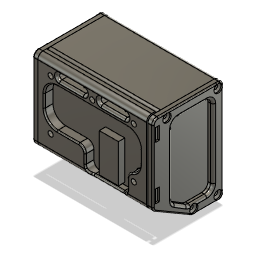
ToolheadExtensionsV2_Type_B v9 (Autodesk Fusion 360 design; units mm, degrees)
Autodesk Fusion 360 part; units mm, degrees
note: some values were not read from the file. Set by a fixed rule: which sketch regions a step uses.
sketch "Sketch1" plane through (0, 0, 0) normal (1, 0, 0) x (0, 0, -1) in component "Head"
  line L0 (0, 0) -> (0, 80)
  line L1 (0, 0) -> (-24, 0)
  line L2 (0, 80) -> (-48, 80)
  line L3 (-48, 80) -> (-48, 14)
  line L4 (-48, 14) -> (-24, 0)
  dimension "d1" = 80
  dimension "d2" = 24
  dimension "d3" = 48
  dimension "d4" = 66
  constraint coincident L0.start L1.start
  constraint vertical L0
  constraint perpendicular L0 L1
  constraint perpendicular L0 L2
  constraint perpendicular L2 L3
  measures "d1" distance of L0.start L0.end
  measures "d2" distance of L0.start L1.end
  measures "d3" distance of L0.end L2.end
  measures "d4" distance of L2.end L3.end
extrude "Extrude1" add sketch "Sketch1" along normal blind 86 makes body 1 in component "Head"
fillet "Fillet1" radius 3 5 edges at (43, 14, 48) (43, 0, 24) (43, 0, 0) (43, 80, 48) (43, 80, 0) on bodies 1 in component "Head"
sketch "Sketch2" plane through (0, 0, 0) normal (-1, 0, 0) x (0, 0, 1) in component "Head"
  arc A0 (3, 80) -> (0, 77) centre (3, 77) ccw
  line L0 (0, 77) -> (0, 3)
  arc A1 (0, 3) -> (3, 0) centre (3, 3) ccw
  line L1 (3, 0) -> (23.188953, 0)
  arc A2 (23.188953, 0) -> (24.700566, 0.408663) centre (23.188953, 3) ccw
  line L2 (24.700566, 0.408663) -> (46.511613, 13.131774)
  arc A3 (46.511613, 13.131774) -> (48, 15.723111) centre (45, 15.723111) ccw
  line L3 (48, 15.723111) -> (48, 77)
  arc A4 (48, 77) -> (45, 80) centre (45, 77) ccw
  line L4 (45, 80) -> (3, 80)
  line L5 (3, 77) -> (4, 77)
  line L6 (4, 77) -> (4, 76)
  line L7 (4, 76) -> (3, 76)
  line L8 (3, 76) -> (3, 77)
  line L9 (4, 76) -> (44, 76)
  line L10 (45, 77) -> (44, 77)
  line L11 (44, 77) -> (44, 76)
  line L12 (44, 76) -> (45, 76)
  line L13 (45, 76) -> (45, 77)
  line L14 (3, 3) -> (4, 3)
  line L15 (4, 3) -> (4, 4)
  line L16 (4, 4) -> (3, 4)
  line L17 (3, 4) -> (3, 3)
  line L18 (4, 4) -> (4, 76)
  line L19 (4, 4) -> (23, 4)
  line L20 (44, 76) -> (44, 16)
  circle A5 centre (4, 76) radius 1.5
  circle A6 centre (44, 76) radius 1.5
  circle A7 centre (23, 4) radius 1.5
  circle A8 centre (4, 4) radius 1.5
  dimension "d11" = 1
  dimension "d12" = 1
  dimension "d13" = 40
  dimension "d14" = 1
  dimension "d15" = 1
  dimension "d16" = 19
  dimension "d17" = 60
  dimension "d18" = 3
  dimension "d19" = 3
  dimension "d21" = 3
  dimension "d22" = 3
  constraint horizontal L5
  constraint vertical L6
  constraint horizontal L7
  constraint vertical L8
  constraint coincident A0.centre L5.start
  constraint perpendicular L6 L9
  constraint horizontal L10
  constraint vertical L11
  constraint horizontal L12
  constraint vertical L13
  constraint coincident A4.centre L10.start
  constraint horizontal L14
  constraint vertical L15
  constraint horizontal L16
  constraint vertical L17
  constraint coincident A1.centre L14.start
  constraint perpendicular L15 L19
  constraint perpendicular L9 L20
  constraint coincident L6.end L7.start
  constraint coincident L9.end L11.end
  constraint coincident L19.end A7.centre
  constraint coincident L15.end L16.start
  measures "d11" distance of A0.centre L5.end
  measures "d12" distance of A0.centre L7.end
  measures "d13" distance of L6.end L9.end
  measures "d14" distance of A1.centre L14.end
  measures "d15" distance of A1.centre L16.end
  measures "d16" distance of L15.end L19.end
  measures "d17" distance of L9.end L20.end
  measures "d18" diameter of A5
  measures "d19" diameter of A6
  measures "d21" diameter of A7
  measures "d22" diameter of A8
extrude "Extrude2" cut sketch "Sketch2" against normal blind 86 contours L9 L18 A5 | L9 L18 A5 | L5 L6 L7 L8 | L10 L11 L12 L13 | L9 L20 A6 | L9 L20 A6 | L14 L15 L16 L17 | L18 L19 A8 | L18 L19 A8 | A7 picked at (4.370476, 76.669113) picked at (4.875443, 75.521972) picked at (3.666667, 76.333333) picked at (44.333333, 76.333333) picked at (44.660764, 75.622125) picked at (43.065438, 75.651426) picked at (3.333333, 3.666667) picked at (4.370476, 3.330887) picked at (4.705305, 4.705305) picked at (22.804781, 5.044492) bodies 1 in component "Head"
sketch "Sketch1 (2)" plane through (0, 0, 0) normal (-1, 0, 0) x (0, 0, 1) in component "SideLeft"
  circle A0 centre (4, 4) radius 1.5
  circle A1 centre (44, 76) radius 1.5
  circle A2 centre (23, 4) radius 1.5
  circle A3 centre (4, 76) radius 1.5
  arc A4 (3, 80) -> (0, 77) centre (3, 77) ccw
  line L0 (0, 77) -> (0, 3)
  arc A5 (0, 3) -> (3, 0) centre (3, 3) ccw
  line L1 (3, 0) -> (23.188953, 0)
  arc A6 (23.188953, 0) -> (24.700566, 0.408663) centre (23.188953, 3) ccw
  line L2 (24.700566, 0.408663) -> (46.511613, 13.131774)
  arc A7 (46.511613, 13.131774) -> (48, 15.723111) centre (45, 15.723111) ccw
  line L3 (48, 15.723111) -> (48, 77)
  arc A8 (48, 77) -> (45, 80) centre (45, 77) ccw
  line L4 (45, 80) -> (3, 80)
  line L5 (4, 76) -> (8, 76)
  line L6 (8, 76) -> (8, 72)
  line L7 (8, 72) -> (4, 72)
  line L8 (4, 72) -> (4, 76)
  line L9 (44, 76) -> (40, 76)
  line L10 (40, 76) -> (40, 72)
  line L11 (40, 72) -> (44, 72)
  line L12 (44, 72) -> (44, 76)
  line L13 (4, 4) -> (8, 4)
  line L14 (8, 4) -> (8, 8)
  line L15 (8, 8) -> (4, 8)
  line L16 (4, 8) -> (4, 4)
  line L17 (23, 4) -> (23, 8)
  line L18 (44, 16) -> (40, 16)
  line L19 (29.797244, 3.381726) -> (27.10325, 8)
  line L20 (27.10325, 8) -> (40, 16)
  line L21 (40, 72) -> (40, 16)
  line L22 (27.10325, 8) -> (23, 8)
  line L23 (23, 8) -> (8, 8)
  line L24 (8, 72) -> (8, 8)
  line L25 (8, 72) -> (40, 72)
  dimension "d33" = 4
  dimension "d34" = 4
  dimension "d35" = 4
  dimension "d36" = 4
  dimension "d37" = 4
  dimension "d38" = 4
  dimension "d39" = 4
  dimension "d40" = 4
  constraint horizontal L5
  constraint vertical L6
  constraint horizontal L7
  constraint vertical L8
  constraint coincident A3.centre L5.start
  constraint horizontal L9
  constraint vertical L10
  constraint horizontal L11
  constraint vertical L12
  constraint coincident A1.centre L9.start
  constraint horizontal L13
  constraint vertical L14
  constraint horizontal L15
  constraint vertical L16
  constraint coincident A0.centre L13.start
  constraint coincident A2.centre L17.start
  constraint vertical L17
  constraint horizontal L18
  constraint perpendicular L2 L19
  constraint perpendicular L21 L22
  measures "d33" distance of A3.centre L5.end
  measures "d34" distance of A3.centre L7.end
  measures "d35" distance of A1.centre L9.end
  measures "d36" distance of A1.centre L11.end
  measures "d37" distance of A0.centre L13.end
  measures "d38" distance of A0.centre L15.end
  measures "d39" distance of A2.centre L17.end
  measures "d40" distance of L18.start L18.end
extrude "Extrude1'" add sketch "Sketch1 (2)" along normal blind 4 separate body contours A3 L5 L6 L7 L8 | A1 L9 L10 L11 L12 | A0 L13 L14 L15 L16 | A4 L0 A5 L1 A6 L2 A7 L3 A8 L4 picked at (7.087293, 74.396346) picked at (42.396346, 72.912707) picked at (7.087293, 5.603654) picked at (44, 34.57437) makes body 2 in component "SideLeft"
fillet "Fillet1'" radius 5 5 edges at (-2, 8, 8) (-2, 8, 27.10325) (-2, 16, 40) (-2, 72, 40) (-2, 72, 8) on bodies 2 in component "SideLeft"
hole "Hole1" at (-4, 76, 4) direction (1, 0, 0) diameter 6.5 depth 1 tip angle 118 bodies 2 in component "SideLeft"
hole "Hole2" at (-4, 76, 44) direction (1, 0, 0) diameter 6.5 depth 1 tip angle 118 bodies 2 in component "SideLeft"
hole "Hole4" at (-4, 4, 23) direction (1, 0, 0) diameter 6.5 depth 1 tip angle 118 bodies 2 in component "SideLeft"
hole "Hole5" at (-4, 4, 4) direction (1, 0, 0) diameter 6.5 depth 1 tip angle 118 bodies 2 in component "SideLeft"
sketch "Sketch2 (2)" plane through (-4, 0, 0) normal (-1, 0, 0) x (0, 0, 1) in component "SideLeft"
  circle A0 centre (4, 4) radius 3.25
  circle A1 centre (23, 4) radius 3.25
  circle A2 centre (44, 76) radius 3.25
  circle A3 centre (4, 76) radius 3.25
  line L0 (37.635654, 14.533369) -> (28.31406, 8.751079)
  arc A4 (25.678406, 8) -> (28.31406, 8.751079) centre (25.678406, 13) ccw
  line L1 (25.678406, 8) -> (13, 8)
  arc A5 (8, 13) -> (13, 8) centre (13, 13) ccw
  line L2 (8, 13) -> (8, 67)
  arc A6 (13, 72) -> (8, 67) centre (13, 67) ccw
  line L3 (13, 72) -> (35, 72)
  arc A7 (40, 67) -> (35, 72) centre (35, 67) ccw
  line L4 (40, 67) -> (40, 18.78229)
  arc A8 (37.635654, 14.533369) -> (40, 18.78229) centre (35, 18.78229) ccw
  line L5 (45, 80) -> (3, 80)
  arc A9 (3, 80) -> (0, 77) centre (3, 77) ccw
  line L6 (0, 77) -> (0, 3)
  arc A10 (0, 3) -> (3, 0) centre (3, 3) ccw
  line L7 (3, 0) -> (23.188953, 0)
  arc A11 (23.188953, 0) -> (24.700566, 0.408663) centre (23.188953, 3) ccw
  line L8 (24.700566, 0.408663) -> (46.511613, 13.131774)
  arc A12 (46.511613, 13.131774) -> (48, 15.723111) centre (45, 15.723111) ccw
  line L9 (48, 15.723111) -> (48, 77)
  arc A13 (48, 77) -> (45, 80) centre (45, 77) ccw
  line L10 (45, 80) -> (55, 80)
  line L11 (46.511613, 13.131774) -> (55, 18.083333)
  line L12 (55, 18.083333) -> (55, 80)
  dimension "d60" = 10
  constraint coincident L5.start A13.end
  constraint perpendicular L9 L10
  constraint tangent A12 L11
  constraint perpendicular L10 L12
  measures "d60" distance of L5.start L10.end
extrude "Extrude2'" add sketch "Sketch2 (2)" against normal blind 4 contours A12 L9 A13 L10 L11 L12 picked at (52.666667, 58.361111) bodies 2 in component "SideLeft"
fillet "Fillet2" radius 4 2 edges at (-2, 80, 55) (-2, 18.083333, 55) on bodies 2 in component "SideLeft"
sketch "Sketch3" plane through (-4, 0, 0) normal (-1, 0, 0) x (0, 0, 1) in component "SideLeft"
  circle A0 centre (4, 4) radius 3.25
  circle A1 centre (23, 4) radius 3.25
  circle A2 centre (44, 76) radius 3.25
  circle A3 centre (4, 76) radius 3.25
  line L0 (37.635654, 14.533369) -> (28.31406, 8.751079)
  arc A4 (25.678406, 8) -> (28.31406, 8.751079) centre (25.678406, 13) ccw
  line L1 (25.678406, 8) -> (13, 8)
  arc A5 (8, 13) -> (13, 8) centre (13, 13) ccw
  line L2 (8, 13) -> (8, 67)
  arc A6 (13, 72) -> (8, 67) centre (13, 67) ccw
  line L3 (13, 72) -> (35, 72)
  arc A7 (40, 67) -> (35, 72) centre (35, 67) ccw
  line L4 (40, 67) -> (40, 18.78229)
  arc A8 (37.635654, 14.533369) -> (40, 18.78229) centre (35, 18.78229) ccw
  arc A9 (53.015484, 16.925699) -> (55, 20.380815) centre (51, 20.380815) ccw
  line L5 (55, 20.380815) -> (55, 76)
  arc A10 (55, 76) -> (51, 80) centre (51, 76) ccw
  line L6 (51, 80) -> (3, 80)
  arc A11 (3, 80) -> (0, 77) centre (3, 77) ccw
  line L7 (0, 77) -> (0, 3)
  arc A12 (0, 3) -> (3, 0) centre (3, 3) ccw
  line L8 (3, 0) -> (23.188953, 0)
  arc A13 (23.188953, 0) -> (24.700566, 0.408663) centre (23.188953, 3) ccw
  line L9 (24.700566, 0.408663) -> (53.015484, 16.925699)
  line L10 (55, 76) -> (53, 76)
  line L11 (53, 76) -> (53, 74)
  line L12 (53, 74) -> (55, 74)
  line L13 (55, 74) -> (55, 76)
  line L14 (53, 74) -> (50, 74)
  line L15 (50, 74) -> (50, 64)
  line L16 (50, 64) -> (53, 64)
  line L17 (53, 64) -> (53, 74)
  line L18 (55, 20.380815) -> (53, 20.380815)
  line L19 (53, 20.380815) -> (53, 22.380815)
  line L20 (53, 22.380815) -> (55, 22.380815)
  line L21 (55, 22.380815) -> (55, 20.380815)
  line L22 (53, 22.380815) -> (50, 22.380815)
  line L23 (50, 22.380815) -> (50, 32.380815)
  line L24 (50, 32.380815) -> (53, 32.380815)
  line L25 (53, 32.380815) -> (53, 22.380815)
  dimension "d65" = 2
  dimension "d66" = 2
  dimension "d67" = 3
  dimension "d68" = 10
  dimension "d69" = 2
  dimension "d70" = 2
  dimension "d71" = 3
  dimension "d72" = 10
  constraint horizontal L10
  constraint vertical L11
  constraint horizontal L12
  constraint vertical L13
  constraint coincident L5.end A10.start
  constraint horizontal L14
  constraint vertical L15
  constraint horizontal L16
  constraint vertical L17
  constraint horizontal L18
  constraint vertical L19
  constraint horizontal L20
  constraint vertical L21
  constraint horizontal L22
  constraint vertical L23
  constraint horizontal L24
  constraint vertical L25
  measures "d65" distance of L5.end L10.end
  measures "d66" distance of L5.end L12.end
  measures "d67" distance of L11.end L14.end
  measures "d68" distance of L11.end L16.end
extrude "Extrude3" cut sketch "Sketch3" against normal blind 4 contours L22 L23 L24 L25 | L14 L15 L16 L17 picked at (51, 25.714148) picked at (51, 67.333333) bodies 2 in component "SideLeft"
fillet "Fillet4" radius 2 10 edges at (-4, 70.535534, 9.464466) (-4, 72, 24) (-4, 70.535534, 38.535534) (-4, 42.891145, 40) (-4, 16.351063, 39.369111) (-4, 11.642224, 32.974857) (-4, 8.191434, 27.048698) (-4, 8, 19.339203) (-4, 9.464466, 9.464466) (-4, 40, 8) on bodies 2 in component "SideLeft"
fillet "Fillet5" radius 1 10 edges at (-4, 78.828427, 53.828427) (-4, 80, 27) (-4, 79.12132, 0.87868) (-4, 40, 0) (-4, 0.87868, 0.87868) (-4, 0, 13.094476) (-4, 0.103967, 23.971893) (-4, 8.667181, 38.858025) (-4, 18.388572, 54.468569) (-4, 48.190407, 55) on bodies 2 in component "SideLeft"
ref_plane "WorkPlane1" through (43, 40, 24) normal (1, 0, 0) x (0, 0, -1)
mirror "MirrorComponent1" about plane through (0, 0, 0) normal (0, 0, 1) of bodies 2 makes body 3 in component "SideLeft(Mirror)"
sketch "Sketch1 (3)" plane through (0, 0, 0) normal (1, 0, 0) x (0, 0, -1) in component "Front_A"
  line L0 (-53, 74) -> (-50, 74)
  line L1 (-50, 74) -> (-50, 64)
  line L2 (-50, 64) -> (-53, 64)
  line L3 (-53, 64) -> (-53, 74)
  line L4 (-50, 32.380815) -> (-50, 22.380815)
  line L5 (-50, 22.380815) -> (-53, 22.380815)
  line L6 (-53, 22.380815) -> (-53, 32.380815)
  line L7 (-53, 32.380815) -> (-50, 32.380815)
  arc A0 (-55, 20.380815) -> (-53.015484, 16.925699) centre (-51, 20.380815) ccw
  line L8 (-53.015484, 16.925699) -> (-24.700566, 0.408663)
  arc A1 (-24.700566, 0.408663) -> (-23.188953, 0) centre (-23.188953, 3) ccw
  line L9 (-23.188953, 0) -> (-3, 0)
  arc A2 (-3, 0) -> (0, 3) centre (-3, 3) ccw
  line L10 (0, 3) -> (0, 77)
  arc A3 (0, 77) -> (-3, 80) centre (-3, 77) ccw
  line L11 (-3, 80) -> (-51, 80)
  arc A4 (-51, 80) -> (-55, 76) centre (-51, 76) ccw
  line L12 (-55, 76) -> (-55, 20.380815)
  circle A5 centre (-4, 76) radius 1.5
  arc A6 (-40, 18.78229) -> (-37.635654, 14.533369) centre (-35, 18.78229) ccw
  line L13 (-40, 18.78229) -> (-40, 67)
  arc A7 (-35, 72) -> (-40, 67) centre (-35, 67) ccw
  line L14 (-35, 72) -> (-13, 72)
  arc A8 (-8, 67) -> (-13, 72) centre (-13, 67) ccw
  line L15 (-8, 67) -> (-8, 13)
  arc A9 (-13, 8) -> (-8, 13) centre (-13, 13) ccw
  line L16 (-13, 8) -> (-25.678406, 8)
  arc A10 (-28.31406, 8.751079) -> (-25.678406, 8) centre (-25.678406, 13) ccw
  line L17 (-28.31406, 8.751079) -> (-37.635654, 14.533369)
  circle A11 centre (-44, 76) radius 1.5
  circle A12 centre (-23, 4) radius 1.5
  circle A13 centre (-4, 4) radius 1.5
  line L18 (-51, 80) -> (-48, 80)
  line L19 (-48, 80) -> (-48, 14)
  dimension "d75" = 3
  constraint coincident L11.end A4.start
  constraint parallel L11 L18
  constraint coincident L8 L19.end
  constraint perpendicular L18 L19
  measures "d75" distance of L11.end L18.end
extrude "Extrude1''" add sketch "Sketch1 (3)" along normal blind 85 separate body contours L0 L1 L2 L3 | L4 L5 L6 L7 | A0 L8 L11 A4 L12 L18 L19 picked at (-51, 67.333333) picked at (-52, 25.714148) picked at (-50.338495, 17.768838) makes body 4 in component "Front_A"
extrude "Extrude2''" add sketch "Sketch1 (3)" against normal blind 4 contours L0 L1 L2 L3 | L4 L5 L6 L7 picked at (-51, 67.333333) picked at (-52, 25.714148) bodies 4 in component "Front_A"
sketch "Sketch2 (3)" plane through (85, 0, 0) normal (1, 0, 0) x (0, 0, -1) in component "Front_A"
  arc A0 (-51, 80) -> (-55, 76) centre (-51, 76) ccw
  line L0 (-55, 76) -> (-55, 20.380815)
  arc A1 (-55, 20.380815) -> (-53.015484, 16.925699) centre (-51, 20.380815) ccw
  line L1 (-53.015484, 16.925699) -> (-48, 14)
  line L2 (-48, 14) -> (-48, 80)
  line L3 (-48, 80) -> (-51, 80)
  line L4 (-55, 76) -> (-53, 76)
  line L5 (-53, 76) -> (-53, 74)
  line L6 (-53, 74) -> (-55, 74)
  line L7 (-55, 74) -> (-55, 76)
  line L8 (-53, 74) -> (-50, 74)
  line L9 (-50, 74) -> (-50, 64)
  line L10 (-50, 64) -> (-53, 64)
  line L11 (-53, 64) -> (-53, 74)
  line L12 (-55, 20.380815) -> (-53, 20.380815)
  line L13 (-53, 20.380815) -> (-53, 22.380815)
  line L14 (-53, 22.380815) -> (-55, 22.380815)
  line L15 (-55, 22.380815) -> (-55, 20.380815)
  line L16 (-53, 22.380815) -> (-50, 22.380815)
  line L17 (-50, 22.380815) -> (-50, 32.380815)
  line L18 (-50, 32.380815) -> (-53, 32.380815)
  line L19 (-53, 32.380815) -> (-53, 22.380815)
  dimension "d80" = 2
  dimension "d81" = 2
  dimension "d82" = 3
  dimension "d83" = 10
  dimension "d84" = 2
  dimension "d85" = 2
  dimension "d86" = 3
  dimension "d87" = 10
  constraint horizontal L4
  constraint vertical L5
  constraint horizontal L6
  constraint vertical L7
  constraint coincident A0.end L0.start
  constraint horizontal L8
  constraint vertical L9
  constraint horizontal L10
  constraint vertical L11
  constraint horizontal L12
  constraint vertical L13
  constraint horizontal L14
  constraint vertical L15
  constraint horizontal L16
  constraint vertical L17
  constraint horizontal L18
  constraint vertical L19
  measures "d80" distance of A0.end L4.end
  measures "d81" distance of A0.end L6.end
  measures "d82" distance of L5.end L8.end
  measures "d83" distance of L5.end L10.end
extrude "Extrude3'" add sketch "Sketch2 (3)" along normal blind 4 contours L8 L9 L10 L11 | L16 L17 L18 L19 picked at (-51, 67.333333) picked at (-52, 29.047481) bodies 4 in component "Front_A"
move_face "OffsetFaces1" offset -0.2 1 faces at (28.333333, 58, 48) on bodies 4 in component "Front_A"
move_face "OffsetFaces2" offset -0.3 16 faces at (-2.666667, 74, 51) (-1.333333, 70.666667, 50) (-1.333333, 67.333333, 53) (-1.333333, 64, 51) (-2.666667, 25.714148, 53) (-1.333333, 22.380815, 51) (-2.666667, 25.714148, 50) (-1.333333, 32.380815, 52) (87.666667, 74, 51) (86.333333, 67.333333, 53) (86.333333, 29.047481, 53) (87.666667, 32.380815, 52) (86.333333, 70.666667, 50) (86.333333, 64, 51) (86.333333, 22.380815, 52) (86.333333, 25.714148, 50) on bodies 4 in component "Front_A"
sketch "Sketch3 (2)" plane through (0, 0, 55) normal (0, 0, 1) x (1, 0, 0) in component "Front_A"
  line L0 (0, 76) -> (0, 20.380815)
  line L1 (0, 20.380815) -> (85, 20.380815)
  line L2 (85, 20.380815) -> (85, 76)
  line L3 (85, 76) -> (0, 76)
  line L4 (0, 76) -> (10, 76)
  line L5 (10, 76) -> (10, 70)
  line L6 (10, 70) -> (0, 70)
  line L7 (0, 70) -> (0, 76)
  line L8 (10, 70) -> (42.5, 70)
  line L9 (42.5, 70) -> (75, 70)
  line L10 (10, 70) -> (10, 30.765)
  line L11 (10, 30.765) -> (42.5, 30.765)
  line L12 (42.5, 30.765) -> (75, 30.765)
  circle A0 centre (10, 30.765) radius 2
  circle A1 centre (42.5, 30.765) radius 2
  circle A2 centre (75, 30.765) radius 2
  circle A3 centre (75, 70) radius 2
  circle A4 centre (42.5, 70) radius 2
  circle A5 centre (10, 70) radius 2
  dimension "d92" = 10
  dimension "d93" = 6
  dimension "d94" = 32.5
  dimension "d95" = 32.5
  dimension "d96" = 39.235
  dimension "d97" = 32.5
  dimension "d98" = 32.5
  dimension "d99" = 4
  dimension "d100" = 4
  dimension "d101" = 4
  dimension "d102" = 4
  dimension "d103" = 4
  dimension "d104" = 4
  constraint horizontal L4
  constraint vertical L5
  constraint horizontal L6
  constraint vertical L7
  constraint coincident L0.start L3.end
  constraint perpendicular L5 L8
  constraint parallel L8 L9
  constraint perpendicular L6 L10
  constraint perpendicular L10 L11
  constraint horizontal L12
  constraint coincident L10.end L11.start
  constraint coincident L11.end L12.start
  constraint coincident L12.end A2.centre
  constraint coincident L9.end A3.centre
  constraint coincident L8.end L9.start
  constraint coincident L5.end L6.start
  measures "d92" distance of L0.start L4.end
  measures "d93" distance of L0.start L6.end
  measures "d94" distance of L5.end L8.end
  measures "d95" distance of L8.end L9.end
  measures "d96" distance of L5.end L10.end
  measures "d97" distance of L10.end L11.end
  measures "d98" distance of L11.end L12.end
  measures "d99" diameter of A0
  measures "d100" diameter of A1
  measures "d101" diameter of A2
  measures "d102" diameter of A3
  measures "d103" diameter of A4
  measures "d104" diameter of A5
extrude "Extrude4" cut sketch "Sketch3 (2)" against normal blind 6.8 contours L5 L6 A5 | L6 L10 A5 | L5 L8 A5 | L8 L10 A5 | L8 L9 A4 | L8 L9 A4 | L10 L11 A0 | L10 L11 A0 | L11 L12 A1 | L11 L12 A1 | A2 | A3 picked at (9.202999, 71.064669) picked at (8.673452, 69.905123) picked at (11.326548, 70.094877) picked at (11.299543, 69.717302) picked at (41.923106, 71.197933) picked at (41.174113, 69.900638) picked at (10.940407, 31.705407) picked at (11.326118, 30.66718) picked at (41.595639, 31.739669) picked at (41.174113, 30.665638) picked at (73.50946, 30.665638) picked at (75.41566, 69.280056) bodies 4 in component "Front_A"
sketch "Sketch4" plane through (0, 0, 55) normal (0, 0, 1) x (1, 0, 0) in component "Front_A"
  circle A0 centre (75, 30.765) radius 2
  circle A1 centre (10, 70) radius 2
  circle A2 centre (42.5, 30.765) radius 2
  circle A3 centre (75, 70) radius 2
  circle A4 centre (42.5, 70) radius 2
  circle A5 centre (10, 30.765) radius 2
  line L0 (0, 76) -> (0, 20.380815)
  line L1 (0, 20.380815) -> (85, 20.380815)
  line L2 (85, 20.380815) -> (85, 76)
  line L3 (85, 76) -> (0, 76)
  line L4 (10, 30.765) -> (10, 70)
  line L5 (10, 50.3825) -> (5, 50.3825)
  line L6 (5, 50.3825) -> (5, 65.3825)
  line L7 (75, 30.765) -> (75, 70)
  line L8 (75, 50.3825) -> (80, 50.3825)
  line L9 (80, 50.3825) -> (80, 35.3825)
  line L10 (80, 35.3825) -> (5, 35.3825)
  line L11 (5, 35.3825) -> (5, 65.3825)
  line L12 (5, 65.3825) -> (80, 65.3825)
  line L13 (80, 65.3825) -> (80, 35.3825)
  dimension "d107" = 5
  dimension "d108" = 15
  dimension "d109" = 5
  dimension "d110" = 15
  constraint coincident A5.centre L4.start
  constraint coincident A1.centre L4.end
  constraint midpoint L4 L5.start
  constraint perpendicular L4 L5
  constraint perpendicular L5 L6
  constraint coincident A0.centre L7.start
  constraint coincident A3.centre L7.end
  constraint midpoint L7 L8.start
  constraint perpendicular L7 L8
  constraint perpendicular L8 L9
  constraint horizontal L10
  constraint vertical L11
  constraint horizontal L12
  constraint vertical L13
  measures "d107" distance of L5.start L5.end
  measures "d108" distance of L5.end L6.end
  measures "d109" distance of L8.start L8.end
  measures "d110" distance of L8.end L9.end
extrude "Extrude5" cut sketch "Sketch4" against normal blind 6.8 contours L4 L5 L10 L11 | L4 L7 L10 L12 | L4 L5 L6 L11 L12 | L7 L8 L9 L10 L13 | L7 L8 L12 L13 picked at (8.333333, 40.3825) picked at (31.666667, 60.3825) picked at (8.333333, 55.3825) picked at (76.666667, 45.3825) picked at (76.666667, 60.3825) bodies 4 in component "Front_A"
fillet "Fillet1''" radius 10 4 edges at (5, 35.3825, 51.6) (80, 35.3825, 51.6) (80, 65.3825, 51.6) (5, 65.3825, 51.6) on bodies 4 in component "Front_A"
sketch "Sketch5" plane through (0, 0, 48.2) normal (0, 0, -1) x (-1, 0, 0) in component "Front_A"
  line L0 (-5, 55.3825) -> (-5, 45.3825)
  arc A0 (-15, 35.3825) -> (-5, 45.3825) centre (-15, 45.3825) ccw
  line L1 (-15, 35.3825) -> (-70, 35.3825)
  arc A1 (-80, 45.3825) -> (-70, 35.3825) centre (-70, 45.3825) ccw
  line L2 (-80, 45.3825) -> (-80, 55.3825)
  arc A2 (-70, 65.3825) -> (-80, 55.3825) centre (-70, 55.3825) ccw
  line L3 (-70, 65.3825) -> (-15, 65.3825)
  arc A3 (-5, 55.3825) -> (-15, 65.3825) centre (-15, 55.3825) ccw
  circle A4 centre (-75, 30.765) radius 2
  circle A5 centre (-10, 70) radius 2
  circle A6 centre (-42.5, 30.765) radius 2
  circle A7 centre (-75, 70) radius 2
  circle A8 centre (-42.5, 70) radius 2
  circle A9 centre (-10, 30.765) radius 2
  line L4 (0, 14.116667) -> (0, 80)
  line L5 (0, 80) -> (-85, 80)
  line L6 (-85, 80) -> (-85, 14.116667)
  line L7 (-85, 14.116667) -> (0, 14.116667)
  circle A10 centre (-75, 70) radius 3.25
  line L8 (-75, 70) -> (-77.5, 70)
  line L9 (-75, 70) -> (-72.5, 70)
  line L10 (-77.5, 70) -> (-77.5, 72.076656)
  line L11 (-77.5, 70) -> (-77.5, 67.923344)
  line L12 (-72.5, 70) -> (-72.5, 67.923344)
  line L13 (-72.5, 70) -> (-72.5, 70.176419)
  line L14 (-72.5, 70.176419) -> (-72.5, 72.076656)
  circle A11 centre (-42.5, 70) radius 3.25
  line L15 (-42.5, 70) -> (-40, 70)
  line L16 (-42.5, 70) -> (-45, 70)
  circle A12 centre (-42.5, 70) radius 2
  line L17 (-40, 70.176419) -> (-40, 72.076656)
  line L18 (-40, 70) -> (-40, 67.923344)
  line L19 (-45, 70) -> (-45, 67.923344)
  line L20 (-40, 70) -> (-40, 70.176419)
  line L21 (-45, 70) -> (-45, 72.076656)
  circle A13 centre (-10, 70) radius 3.25
  line L22 (-10, 70) -> (-7.5, 70)
  line L23 (-10, 70) -> (-12.5, 70)
  circle A14 centre (-10, 70) radius 2
  line L24 (-7.5, 70.176419) -> (-7.5, 72.076656)
  line L25 (-7.5, 70) -> (-7.5, 67.923344)
  line L26 (-12.5, 70) -> (-12.5, 67.923344)
  line L27 (-7.5, 70) -> (-7.5, 70.176419)
  line L28 (-12.5, 70) -> (-12.5, 72.076656)
  circle A15 centre (-75, 30.765) radius 3.25
  line L29 (-75, 30.765) -> (-72.5, 30.765)
  line L30 (-75, 30.765) -> (-77.5, 30.765)
  circle A16 centre (-75, 30.765) radius 2
  line L31 (-72.5, 30.941419) -> (-72.5, 32.841656)
  line L32 (-72.5, 30.765) -> (-72.5, 28.688344)
  line L33 (-77.5, 30.765) -> (-77.5, 28.688344)
  line L34 (-72.5, 30.765) -> (-72.5, 30.941419)
  line L35 (-77.5, 30.765) -> (-77.5, 32.841656)
  circle A17 centre (-42.5, 30.765) radius 3.25
  line L36 (-42.5, 30.765) -> (-40, 30.765)
  line L37 (-42.5, 30.765) -> (-45, 30.765)
  circle A18 centre (-42.5, 30.765) radius 2
  line L38 (-40, 30.941419) -> (-40, 32.841656)
  line L39 (-40, 30.765) -> (-40, 28.688344)
  line L40 (-45, 30.765) -> (-45, 28.688344)
  line L41 (-40, 30.765) -> (-40, 30.941419)
  line L42 (-45, 30.765) -> (-45, 32.841656)
  circle A19 centre (-10, 30.765) radius 3.25
  line L43 (-10, 30.765) -> (-7.5, 30.765)
  line L44 (-10, 30.765) -> (-12.5, 30.765)
  circle A20 centre (-10, 30.765) radius 2
  line L45 (-7.5, 30.941419) -> (-7.5, 32.841656)
  line L46 (-7.5, 30.765) -> (-7.5, 28.688344)
  line L47 (-12.5, 30.765) -> (-12.5, 28.688344)
  line L48 (-7.5, 30.765) -> (-7.5, 30.941419)
  line L49 (-12.5, 30.765) -> (-12.5, 32.841656)
  dimension "d115" = 6.5
  dimension "d116" = 2.5
  dimension "d117" = 2.5
  dimension "d120" = 65
  dimension "d121" = -39.235
  constraint concentric A7 A10
  constraint coincident A7.centre A10.centre
  constraint horizontal L8
  constraint parallel L8 L9
  constraint perpendicular L8 L10
  constraint perpendicular L8 L11
  constraint perpendicular L9 L12
  constraint perpendicular L9 L13
  constraint perpendicular L9 L14
  measures "d115" diameter of A10
  measures "d116" distance of A7.centre L8.end
  measures "d117" distance of A7.centre L9.end
extrude "Extrude6" cut sketch "Sketch5" against normal blind 3 contours A4 A15 L29 L30 A16 L32 L33 | A4 A15 L29 L30 A16 L31 L34 L35 | A5 A13 L22 L23 A14 L25 L26 | A5 A13 L22 L23 A14 L24 L27 L28 | A6 A17 L36 L37 A18 L39 L40 | A6 A17 L36 L37 A18 L38 L41 L42 | A7 A10 L8 L9 L11 L12 | A7 A10 L8 L9 L10 L13 L14 | A8 A11 L15 L16 A12 L18 L19 | A8 A11 L15 L16 A12 L17 L20 L21 | A9 A19 L43 L44 A20 L46 L47 | A9 A19 L43 L44 A20 L45 L48 L49 picked at (-72.696285, 29.876278) picked at (-72.732687, 31.805281) picked at (-7.696285, 69.111278) picked at (-7.732687, 71.040281) picked at (-40.196285, 29.876278) picked at (-40.232687, 31.805281) picked at (-72.696285, 69.111278) picked at (-72.732687, 71.040281) picked at (-40.196285, 69.111278) picked at (-40.232687, 71.040281) picked at (-12.303715, 29.876278) picked at (-7.732687, 31.805281) bodies 4 in component "Front_A"
sketch "Sketch6" plane through (0, 0, 55) normal (0, 0, 1) x (1, 0, 0) in component "Front_A"
  line L0 (0, 76) -> (0, 20.380815)
  line L1 (0, 20.380815) -> (85, 20.380815)
  line L2 (85, 20.380815) -> (85, 76)
  line L3 (85, 76) -> (0, 76)
  circle A0 centre (10, 30.765) radius 2
  circle A1 centre (42.5, 70) radius 2
  circle A2 centre (75, 70) radius 2
  circle A3 centre (42.5, 30.765) radius 2
  circle A4 centre (10, 70) radius 2
  circle A5 centre (75, 30.765) radius 2
  line L4 (0, 76) -> (15, 76)
  line L5 (15, 76) -> (15, 74)
  line L6 (40.5, 70) -> (37.5, 70)
  line L7 (44.5, 70) -> (47.5, 70)
  line L8 (85, 76) -> (70, 76)
  line L9 (70, 76) -> (70, 74)
  line L10 (70, 74) -> (47.5, 74)
  line L11 (47.5, 74) -> (47.5, 70)
  line L12 (47.5, 70) -> (70, 70)
  line L13 (70, 70) -> (70, 74)
  line L14 (37.5, 70) -> (15, 70)
  line L15 (15, 70) -> (15, 74)
  line L16 (15, 74) -> (37.5, 74)
  line L17 (37.5, 74) -> (37.5, 70)
  line L18 (70, 33.3825) -> (70, 38.3825)
  line L19 (70, 33.3825) -> (70, 18.3825)
  line L20 (70, 18.3825) -> (37, 18.3825)
  line L21 (37, 18.3825) -> (37, 38.3825)
  line L22 (37, 38.3825) -> (70, 38.3825)
  line L23 (5, 45.3825) -> (5, 55.3825)
  arc A6 (15, 65.3825) -> (5, 55.3825) centre (15, 55.3825) ccw
  line L24 (15, 65.3825) -> (70, 65.3825)
  arc A7 (80, 55.3825) -> (70, 65.3825) centre (70, 55.3825) ccw
  line L25 (80, 55.3825) -> (80, 45.3825)
  arc A8 (70, 35.3825) -> (80, 45.3825) centre (70, 45.3825) ccw
  line L26 (70, 35.3825) -> (15, 35.3825)
  arc A9 (5, 45.3825) -> (15, 35.3825) centre (15, 45.3825) ccw
  dimension "d139" = 15
  dimension "d140" = 2
  dimension "d141" = 3
  dimension "d142" = 3
  dimension "d143" = 15
  dimension "d144" = 2
  dimension "d169" = 5
  dimension "d170" = 15
  dimension "d171" = 33
  constraint coincident L0.start L3.end
  constraint perpendicular L0 L4
  constraint perpendicular L4 L5
  constraint coincident A1 L6.start
  constraint perpendicular L5 L6
  constraint coincident A1 L7.start
  constraint horizontal L7
  constraint coincident L2.end L3.start
  constraint perpendicular L2 L8
  constraint perpendicular L8 L9
  constraint horizontal L10
  constraint vertical L11
  constraint horizontal L12
  constraint vertical L13
  constraint horizontal L14
  constraint vertical L15
  constraint horizontal L16
  constraint vertical L17
  constraint perpendicular L1 L19
  constraint perpendicular L19 L20
  constraint perpendicular L18 L22
  measures "d139" distance of L0.start L4.end
  measures "d140" distance of L4.end L5.end
  measures "d141" distance of L6.start L6.end
  measures "d142" distance of L7.start L7.end
  measures "d143" distance of L2.end L8.end
  measures "d144" distance of L8.end L9.end
  measures "d169" distance of L18.start L18.end
  measures "d170" distance of L18.start L19.end
  measures "d171" distance of L19.end L20.end
extrude "Extrude7" cut sketch "Sketch6" against normal blind 6.8 contours L1 L18 L19 L21 L26 | L1 L19 L20 L21 | L14 L15 L16 L17 | L18 L21 L22 L26 | L10 L11 L12 L13 picked at (61.470382, 27.979601) picked at (48, 19.71471) picked at (22.5, 72.666667) picked at (48, 36.3825) picked at (55, 72.666667) bodies 4 in component "Front_A"
fillet "Fillet3" radius 5 4 edges at (37, 18.3825, 51.332537) (70, 18.3825, 51.332537) (37, 35.3825, 51.6) (70, 35.3825, 51.6) on bodies 4 in component "Front_A"
fillet "Fillet4'" radius 2 8 edges at (15, 70, 51.6) (15, 74, 51.6) (37.5, 74, 51.6) (37.5, 70, 51.6) (47.5, 70, 51.6) (47.5, 74, 51.6) (70, 74, 51.6) (70, 70, 51.6) on bodies 4 in component "Front_A"
sketch "Sketch3 (3)" plane through (0, 0, 48) normal (0, 0, 1) x (1, 0, 0) in component "Head"
  line L0 (86, 77) -> (0, 77)
  line L1 (0, 77) -> (0, 15.723111)
  line L2 (0, 15.723111) -> (86, 15.723111)
  line L3 (86, 15.723111) -> (86, 77)
  line L4 (86, 77) -> (86, 80)
  line L5 (86, 80) -> (61, 80)
  line L6 (61, 80) -> (61, 50)
  line L7 (61, 50) -> (86, 50)
  line L8 (86, 50) -> (86, 80)
  line L9 (61, 50) -> (46, 50)
  line L10 (46, 50) -> (46, 20)
  line L11 (46, 20) -> (61, 20)
  line L12 (61, 20) -> (61, 50)
  dimension "d157" = 3
  dimension "d158" = 25
  dimension "d159" = 30
  dimension "d160" = 15
  dimension "d161" = 30
  constraint coincident L0.start L3.end
  constraint perpendicular L0 L4
  constraint horizontal L5
  constraint vertical L6
  constraint horizontal L7
  constraint vertical L8
  constraint horizontal L9
  constraint vertical L10
  constraint horizontal L11
  constraint vertical L12
  measures "d157" distance of L0.start L4.end
  measures "d158" distance of L4.end L5.end
  measures "d159" distance of L4.end L7.end
  measures "d160" distance of L6.end L9.end
  measures "d161" distance of L6.end L11.end
extrude "Extrude3''" add sketch "Sketch3 (3)" along normal blind 5 contours L9 L10 L11 L12 picked at (51, 40) bodies 1 in component "Head"
sketch "Sketch4 (2)" plane through (0, 0, 0) normal (0, -1, 0) x (1, 0, 0) in component "Head"
  line L0 (0, 3) -> (86, 3)
  line L1 (86, 3) -> (86, 23.188953)
  line L2 (86, 23.188953) -> (0, 23.188953)
  line L3 (0, 23.188953) -> (0, 3)
  line L4 (86, 23.188953) -> (61, 23.188953)
  line L5 (61, 23.188953) -> (53.5, 23.188953)
  line L6 (53.5, 23.188953) -> (53.5, 3)
  circle A0 centre (53.5, 13.094476) radius 6
  dimension "d164" = 25
  dimension "d165" = 7.5
  dimension "d166" = 12
  constraint perpendicular L1 L4
  constraint parallel L2 L5
  constraint coincident L0 L6.end
  constraint perpendicular L0 L6
  measures "d166" diameter of A0
extrude "Extrude4'" add sketch "Sketch4 (2)" along normal blind 5 contours L6 A0 | L6 A0 picked at (51.505592, 12.945016) picked at (57.912045, 11.890861) bodies 1 in component "Head"
fillet "Fillet7" radius 1 17 edges at (39.761735, 18.9115, 54.72034) (37.256917, 21.800362, 55) (37, 26.8825, 55) (35.535534, 33.918034, 55) (23.5, 35.3825, 55) (7.928932, 38.311432, 55) (5, 50.3825, 55) (7.928932, 62.453568, 55) (42.5, 65.3825, 55) (77.071068, 62.453568, 55) (80, 50.3825, 55) (78.164966, 39.608997, 55) (70.917517, 34.127116, 55) (70, 27.311432, 55) (69.743083, 21.800362, 55) (67.238265, 18.9115, 54.72034) (53.5, 18.3825, 54.465074) on bodies 4 in component "Front_A"
fillet "Fillet8" radius 2 8 edges at (15, 72, 55) (26.25, 74, 55) (37.5, 72, 55) (26.25, 70, 55) (47.5, 72, 55) (58.75, 74, 55) (70, 72, 55) (58.75, 70, 55) on bodies 4 in component "Front_A"
component "Head" placed x (1, 0, 0) y (0, 1, 0) z (0, 0, 1) at (0, 0, 0)
component "SideLeft" placed x (1, 0, 0) y (0, 1, 0) z (0, 0, 1) at (0, 0, 0)
component "Front_A" placed x (1, 0, 0) y (0, 1, 0) z (0, 0, 1) at (0, 0, 0)
component "SideLeft(Mirror)" placed x (-1, 0, 0) y (0, 1, 0) z (0, 0, -1) at (86, 0, 0)
equation "d165 = ( 15 / 2 ) * 1 mm"
